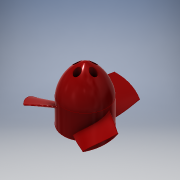
# Autodesk Inventor part: Propeller
Saved by Autodesk Inventor 2017 (Build 210142000, 142)
## iProperties
Created: 2017-08-01
Part Number: Propeller
Material: Generic
Document SubType Name: Modeling
Designer: Thein Lin Aung
Density: 1 g/cm^3
Appearance: Red
Author: Thein Lin Aung
Autodesk Inventor part; units mm, degrees
ref_plane "YZ Plane" through (0, 0, 0) normal (1, 0, 0) x (0, 1, 0)
ref_plane "XY Plane" through (0, 0, 0) normal (0, 0, 1) x (1, 0, 0)
sketch "Sketch1" plane through (0, 0, 0) normal (0, 0, 1) x (1, 0, 0)
  circle A0 centre (0, 0) radius 14.05
  circle A1 centre (0, 0) radius 16.05
  dimension "d0" = 28.1
  dimension "d1" = 2
  constraints: 2 centre point, 1 coincident
  measures "d0" diameter of A0
  measures "d1" radial gap between concentric circles of A1 A0
extrude "Extrusion1" add sketch "Sketch1" along normal blind 18
sketch "Sketch2" plane through (0, 0, 0) normal (1, 0, 0) x (0, 1, 0)
  line L0 (0, -8.4682) -> (0, 50.8092) projected
  line L1 (16.05, 18) -> (16.05, 21.5197) construction
  spline S0 degree 3 poles (16.05, 18) (16.05, 21.5197) (13.0965, 33.8196) (1, 40) knots 1 1 1 1 1.986312 1.986312 1.986312 1.986312
  line L2 (-16.05, 0) -> (16.05, 0) projected
  line L3 (-14.05, 18) -> (14.05, 18) projected
  line L4 (14.05, 0) -> (-14.05, 0) projected
  line L5 (-14.05, 18) -> (14.05, 18) projected
  line L6 (-14.05, 18) -> (14.05, 18) projected
  line L7 (16.05, 18) -> (-16.05, 18) projected
  line L8 (14.05, 18) -> (16.05, 18)
  line L9 (0, 40) -> (0, 18)
  line L10 (16.05, 18) -> (-16.05, 18) projected
  line L11 (0, 18) -> (16.05, 18)
  line L12 (0, 40) -> (1, 40)
  line L13 (16.05, 21.5197) -> (13.0965, 33.8196) construction
  line L14 (13.0965, 33.8196) -> (1, 40) construction
  line L15 (16.05, 0) -> (16.05, 18) projected
  point P0 (0, 0)
  dimension "d6" = 40
  dimension "d7" = 1
  constraints: 8 end point, 2 collinear, 1 horizontal, 1 midpoint, 1 perpendicular, 3 other
  measures "d6" distance between parallel lines of L4 L12
  measures "d7" distance of L9.start L12.end
revolve "Revolution1" add sketch "Sketch2" angle 360 about axis through (0, 0, -10) along (0, 0, 1) separate body contours L0 L12 S0 L7 L3
ref_plane "Work Plane2" through (0, 9.5, 0) normal (0, 1, 0) x (-1, 0, 0)
sketch "Sketch4" plane through (0, 9.5, 0) normal (0, 1, 0) x (-1, 0, 0)
  line L0 (11.891, 18) -> (6.6361, 8.8982) construction
  line L1 (6.6361, 8.8982) -> (-6.6361, 9.1018) construction
  line L2 (-6.6361, 9.1018) -> (-11.891, 0) construction
  spline S0 degree 3 poles (11.891, 18) (6.6361, 8.8982) (-6.6361, 9.1018) (-11.891, 0) knots 1 1 1 1 2 2 2 2 construction
  line L3 (11.891, 18) -> (6.3293, 11.4032) construction
  line L4 (6.3293, 11.4032) -> (-5.2052, 11.5801) construction
  line L5 (-5.2052, 11.5801) -> (-11.891, 0) construction
  spline S1 degree 3 poles (11.891, 18) (6.3293, 11.4032) (-5.2052, 11.5801) (-11.891, 0) knots 1 1 1 1 2 2 2 2
  line L6 (11.891, 18) -> (3.8786, 6.4402) construction
  line L7 (3.8786, 6.4402) -> (-7.3082, 6.6118) construction
  line L8 (-7.3082, 6.6118) -> (-11.891, 0) construction
  spline S2 degree 3 poles (11.891, 18) (3.8786, 6.4402) (-7.3082, 6.6118) (-11.891, 0) knots 1 1 1 1 2 2 2 2
  line L9 (0, -4.4474) -> (0, 22.8408) construction
  line L10 (16.05, 18) -> (-16.05, 18) construction
  line L11 (-16.05, 0) -> (16.05, 0) construction
  line L12 (0, 18) -> (0, 0) construction
  point P0 (9.5932, 15.0042)
  point P1 (0, 9)
  dimension "d29" = 60
  dimension "d50" = 5
  dimension "d51" = 2.5
  constraints: 5 parallel, 4 midpoint, 3 point on line, 2 end point, 1 collinear, 10 other
  measures "d29" angle of L11 L2
  measures "d50" distance between parallel lines of L4 L7
  measures "d51" distance between parallel lines of L4 L1
ref_plane "Work Plane1" through (0, 35, 0) normal (0, 1, 0) x (-1, 0, 0)
sketch "Sketch5" plane through (0, 35, 0) normal (0, 1, 0) x (-1, 0, 0)
  line L0 (16.05, 18) -> (-16.05, 18) construction
  line L1 (-16.05, 0) -> (16.05, 0) construction
  line L2 (-10.3366, 5.2378) -> (-4.7979, 9.116) construction
  line L3 (-4.7979, 9.116) -> (3.6009, 12.1729) construction
  line L4 (16.05, 18) -> (-16.05, 18) construction
  line L5 (3.6009, 12.1729) -> (10.3366, 12.7622) construction
  spline S0 degree 3 poles (-10.3366, 5.2378) (-4.7979, 9.116) (3.6009, 12.1729) (10.3366, 12.7622) knots 1 1 1 1 2 2 2 2
  spline S1 degree 3 poles (11.891, 18) (6.6361, 8.8982) (-6.6361, 9.1018) (-11.891, 0) knots 1 1 1 1 2 2 2 2 construction
  line L6 (-10.3366, 5.2378) -> (10.3366, 12.7622) construction
  line L7 (-10.3366, 5.2378) -> (-3.6009, 5.8271) construction
  line L8 (-3.6009, 5.8271) -> (4.7979, 8.884) construction
  line L9 (4.7979, 8.884) -> (10.3366, 12.7622) construction
  spline S2 degree 3 poles (-10.3366, 5.2378) (-3.6009, 5.8271) (4.7979, 8.884) (10.3366, 12.7622) knots 1 1 1 1 2 2 2 2
  line L10 (0, -3.852) -> (0, 21.852) construction
  point P0 (0, 0)
  point P1 (16.05, 0)
  point P2 (7.834, 11.1743)
  point P3 (-10.8516, 1.2641)
  point P4 (0, 9)
  point P5 (-10.4804, 0)
  dimension "d22" = 30
  dimension "d23" = 3.5
  dimension "TipAngleOfAttact" = 20
  dimension "d31" = 22
  constraints: 2 end point, 2 midpoint, 2 symmetric about line, 1 equal length, 1 parallel, 9 other
  measures "d22" angle of L2 L7
  measures "d23" distance between parallel lines of L3 L8
  measures "TipAngleOfAttact" angle to the sketch x axis of L6
  measures "d31" distance of L2.start L5.end
loft "Loft1" add profiles "Sketch4", "Sketch5" bodies 1
pattern_circular "Circular Pattern1" count 3 over 360 about axis through (0, 0, -10) along (0, 0, 1) of "Loft1" bodies 1
sketch "Sketch7" plane through (0, 0, 0) normal (0, 0, 1) x (1, 0, 0)
  circle A0 centre (0, 0) radius 32.5
  circle A1 centre (0, 0) radius 44.5
  dimension "d37" = 65
  dimension "d38" = 12
  constraints: 2 centre point, 2 coincident
  measures "d37" diameter of A0
  measures "d38" radial gap between concentric circles of A1 A0
extrude "Extrusion5" cut sketch "Sketch7" along normal up to surface (40 mm away) bodies 1
sketch "Sketch8" plane through (0, 0, 0) normal (0, 0, -1) x (-1, 0, 0)
  circle A0 centre (0, 0) radius 14.05 projected
  circle A1 centre (0, 0) radius 14.05
  point P0 (-3.1196, -13.5967)
  point P1 (-10.2153, 9.5)
  constraints: 1 centre point, 1 coincident, 2 other
extrude "Extrusion6" cut sketch "Sketch8" against normal blind 21.7 bodies 1 2
ref_plane "Work Plane3" through (0, 0, 21.7) normal (0, 0, -1) x (-1, 0, 0)
sketch "Sketch9" plane through (0, 0, 21.7) normal (0, 0, -1) x (-1, 0, 0)
  circle A0 centre (0, 0) radius 14.05 projected
extrude "Extrusion7" add sketch "Sketch9" against normal blind 4 bodies 1
sketch "Sketch10" plane through (0, 0, 25.7) normal (0, 0, 1) x (1, 0, 0)
  line L0 (-46.7693, 0) -> (46.7693, 0) projected
  line L1 (0, -36.9152) -> (0, 44.0942) projected
  circle A0 centre (-6, 0) radius 1.25
  point P0 (0, 0)
  dimension "d58" = 2.5
  dimension "d59" = 6
  constraints: 1 centre point, 1 point on line
  measures "d58" diameter of A0
  measures "d59" distance from line of L1 A0.centre
extrude "Extrusion8" cut sketch "Sketch10" along normal through all both and the other way through all bodies 1 2
sketch "Sketch11" plane through (0, 0, 25.7) normal (0, 0, 1) x (1, 0, 0)
  circle A0 centre (-6, 0) radius 1.25 projected
  circle A1 centre (-6, 0) radius 2.4
  point P0 (0, 0)
  dimension "d62" = 4.8
  constraints: 1 centre point, 1 coincident, 1 horizontal alignment, 1 other
  measures "d62" diameter of A1
extrude "Extrusion9" cut sketch "Sketch11" along normal through all bodies 1 2
pattern_circular "Circular Pattern2" count 4 over 360 about axis through (0, 0, -10) along (0, 0, 1) of "Extrusion8", "Extrusion9" bodies 2 1
sketch "Sketch12" plane through (0, 0, 21.7) normal (0, 0, -1) x (-1, 0, 0)
  circle A0 centre (0, 0) radius 1.78
  dimension "d68" = 3.56
  constraints: 1 centre point, 1 coincident
  measures "d68" diameter of A0
extrude "Extrusion10" cut sketch "Sketch12" against normal blind 16.5 bodies 2 1
sketch "Sketch13" plane through (0, 0, 21.7) normal (0, 0, -1) x (-1, 0, 0)
  circle A0 centre (0, 0) radius 4.635
  dimension "d71" = 9.27
  constraints: 1 centre point, 1 coincident
  measures "d71" diameter of A0
extrude "Extrusion11" cut sketch "Sketch13" against normal blind 2.5 bodies 2 1
combine bodies "Combine1" operation type add bodies to combine 1 2
fillet "Fillet2" radius 0.3 6 edges at (11.2023, 20.7976, 2.3206) (12.4101, -20.1003, 2.3206) (-23.6124, -0.6973, 2.3206) (-12.4101, -20.1003, 15.6794) (23.6124, -0.6973, 15.6794) (-11.2023, 20.7976, 15.6794)
sketch "Sketch14" plane through (0, 0, 21.7) normal (0, 0, -1) x (-1, 0, 0)
  circle A0 centre (0, 0) radius 14.05 projected
extrude "Extrusion12" add sketch "Sketch14" along normal blind 0.2 separate body
sketch "Sketch15" plane through (0, 0, 24.2) normal (0, 0, -1) x (-1, 0, 0)
  circle A0 centre (0, 0) radius 1.78 projected
  circle A1 centre (0, 0) radius 4.635 projected
extrude "Extrusion13" add sketch "Sketch15" along normal blind 0.2 contours A0 | A1 bodies 3
sketch "Sketch16" plane through (0, 0, 0) normal (0, 0, -1) x (-1, 0, 0)
  circle A0 centre (0, 0) radius 14.05 projected
extrude "Extrusion14" add sketch "Sketch16" against normal blind 0.2 bodies 3
sketch "Sketch17" plane through (0, 0, 0) normal (0, 1, 0) x (-1, 0, 0)
  line L0 (-14.05, 21.5) -> (14.05, 21.5) projected
  line L1 (14.05, 0) -> (14.05, 21.7) projected
  line L2 (14.05, 17.5) -> (10.6936, 21.5)
  line L3 (0, -4.34) -> (0, 26.04) projected
  point P0 (0, 0)
  dimension "d112" = 40
  dimension "d113" = 4
  constraints: 2 end point, 2 point on line
  measures "d112" angle of L1 L2
  measures "d113" distance from line of L0 L2.start
revolve "Revolution2" add sketch "Sketch17" angle 360 about axis through (0, 0, -10) along (0, 0, 1) bodies 3
equation "\"d51\" = 0.5 * d50"
